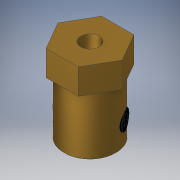
# Autodesk Inventor part: Wheel Coupler
Saved by Autodesk Inventor 2018 (Build 220112000, 112)
## iProperties
Created: 2018-03-28
Part Number: Wheel Coupler
Material: Generic
Document SubType Name: Modeling
Designer: Ajith Thomas
Density: 1 g/cm^3
Appearance: Default
Author: Ajith Thomas
Autodesk Inventor part; units mm, degrees
ref_plane "YZ Plane" through (0, 0, 0) normal (1, 0, 0) x (0, 1, 0)
ref_plane "XZ Plane" through (0, 0, 0) normal (0, 1, 0) x (-1, 0, 0)
sketch "Sketch1" plane through (0, 0, 0) normal (0, 1, 0) x (-1, 0, 0)
  circle A0 centre (0, 0) radius 5.65
  circle A1 centre (0, 0) radius 2.5
  dimension "d0" = 11.3
  dimension "d1" = 5
  constraints: 2 centre point, 2 coincident
  measures "d0" diameter of A0
  measures "d1" diameter of A1
extrude "Extrusion1" add sketch "Sketch1" along normal mid plane 18.1
sketch "Sketch2" plane through (0, 9.05, 0) normal (0, 1, 0) x (1, 0, 0)
  circle A0 centre (0, 0) radius 6 construction
  line L0 (3.4641, 6) -> (6.9282, 0)
  line L1 (6.9282, 0) -> (3.4641, -6)
  line L2 (3.4641, -6) -> (-3.4641, -6)
  line L3 (-3.4641, -6) -> (-6.9282, 0)
  line L4 (-6.9282, 0) -> (-3.4641, 6)
  line L5 (-3.4641, 6) -> (3.4641, 6)
  circle A1 centre (0, 0) radius 5.65 projected
  point P0 (0, 6)
  dimension "d4" = 12
  constraints: 12 end point, 2 coincident, 1 midpoint, 1 vertical alignment, 15 other
extrude "Extrusion2" add sketch "Sketch2" against normal blind 5.5
sketch "Sketch3" plane through (0, 9.05, 0) normal (0, 1, 0) x (1, 0, 0)
  circle A0 centre (0, 0) radius 2
  circle A1 centre (0, 0) radius 2.5 projected
  dimension "d7" = 4
  constraints: 1 centre point, 1 coincident
  measures "d7" diameter of A0
extrude "Extrusion3" add sketch "Sketch3" against normal blind 5.5
ref_plane "Work Plane1" through (4.893, 0, -2.825) normal (0.8660254, 0, -0.5) x (0, 1, 0)
sketch "Sketch4" plane through (4.893, 0, -2.825) normal (0.8660254, 0, -0.5) x (0, 1, 0)
  circle A0 centre (-4.55, 0) radius 2
  line L0 (-9.05, 5.65) -> (-9.05, -5.65) projected
  point P0 (0, 0)
  dimension "d10" = 4
  dimension "d11" = 4.5
  constraints: 1 centre point
  measures "d10" diameter of A0
  measures "d11" distance from line of L0 A0.centre
extrude "Extrusion4" cut sketch "Sketch4" against normal blind 16.6125
chamfer "Chamfer1" distance 0.2 angle 45 2 edges at (5.65, -9.05, 0) (2.5, -9.05, 0)
fillet "Fillet1" radius 0.1 2 edges at (-4.8917, -6.55, 2.8273) (4.8943, -6.55, -2.8227)
fillet_without_effect "Fillet2"
thread "Thread1" size "M4x0.7" class "6H" standard "ANSI Metric M Profile" full length
thread "Thread2" size "M4x0.7" class "6H" standard "ANSI Metric M Profile" full length
sketch "Sketch5" plane through (4.893, 0, -2.825) normal (0.8660254, 0, -0.5) x (0, 1, 0)
  spline S0 degree 5 poles (-2.55, 0) (-2.55, 0.1817) (-2.5708, 0.3632) (-2.6116, 0.5381) (-2.6699, 0.7023) (-2.8134, 1.0061) (-2.8989, 1.1458) (-2.9953, 1.2725) (-3.1005, 1.3863) (-3.4382, 1.6899) (-3.6924, 1.8421) (-3.967, 1.9451) (-4.2528, 1.9984) (-4.7946, 2.0014) (-5.0505, 1.9616) (-5.2985, 1.8818) (-5.5319, 1.7625) (-5.9583, 1.4448) (-6.1506, 1.2458) (-6.317, 1.0081) (-6.4424, 0.7211) (-6.5468, 0.2223) (-6.5645, 0.0253) (-6.5571, -0.1731) (-6.5252, -0.3662) (-6.4219, -0.729) (-6.3503, -0.8991) (-6.2626, -1.0549) (-6.1623, -1.1951) (-5.8146, -1.5907) (-5.5297, -1.7922) (-5.2179, -1.9296) (-4.8859, -1.9993) (-4.2807, -2.0006) (-4.007, -1.954) (-3.7429, -1.8617) (-3.4967, -1.7242) (-3.1533, -1.4403) (-3.0391, -1.3255) (-2.934, -1.1963) (-2.8404, -1.0527) (-2.6828, -0.7379) (-2.6185, -0.567) (-2.5733, -0.3833) (-2.55, -0.1914) (-2.55, 0) knots 0 0 0 0 0 0 0.062286 0.062286 0.062286 0.062286 0.124572 0.124572 0.124572 0.124572 0.249144 0.249144 0.249144 0.249144 0.360428 0.360428 0.360428 0.360428 0.471711 0.471711 0.471711 0.471711 0.538648 0.538648 0.538648 0.538648 0.605585 0.605585 0.605585 0.605585 0.749763 0.749763 0.749763 0.749763 0.868757 0.868757 0.868757 0.868757 0.934378 0.934378 0.934378 0.934378 1 1 1 1 1 1 projected
  point P0 (0, 0)
  constraints: 1 other
extrude "Extrusion5" add sketch "Sketch5" against normal blind 3.7 separate body
chamfer "Chamfer2" distance 0.1 angle 45 1 edges at (4.8943, -6.55, -2.8228)
sketch "Sketch6" plane through (4.893, 0, -2.825) normal (0.8660254, 0, -0.5) x (-0.5, 0, -0.8660254)
  line L0 (0.0058, -6.45) -> (0.0058, -2.65) construction
  line L1 (0.0058, -3.4738) -> (0.9379, -4.0119)
  line L2 (0.9379, -4.0119) -> (0.9379, -5.0881)
  line L3 (0.9379, -5.0881) -> (0.0058, -5.6262)
  line L4 (0.0058, -5.6262) -> (-0.9262, -5.0881)
  line L5 (-0.9262, -5.0881) -> (-0.9262, -4.0119)
  line L6 (-0.9262, -4.0119) -> (0.0058, -3.4738)
  point P0 (0, 0)
  point P1 (0.0058, -4.55)
  constraints: 14 end point, 1 midpoint, 1 point on line, 1 vertical, 1 vertical alignment, 14 other
extrude "Extrusion6" cut sketch "Sketch6" against normal blind 1 bodies 2
body "Solid1"
body "Solid2"
